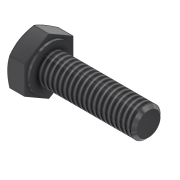
# Autodesk Inventor part: Sechskantschraube ISO 4017-M6x20-8.8
Saved by Autodesk Inventor 2015 (Build 190159000, 159)
## iProperties
Created: 2012-06-21
Part Number: Sechskantschraube ISO 4017-M6x20-8.8
Material: Steel
Document SubType Name: Modeling
Mass: 7.03009 g
Surface Area: 6.76348 cm^2
Volume: 0.895553 cm^3
Density: 7.85 g/cm^3
Appearance: Steel Galvanized 2
Autodesk Inventor part; units mm, degrees
ref_plane "YZ Plane" through (0, 0, 0) normal (1, 0, 0) x (0, 1, 0)
ref_plane "XZ Plane" through (0, 0, 0) normal (0, 1, 0) x (-1, 0, 0)
ref_plane "XY Plane" through (0, 0, 0) normal (0, 0, 1) x (1, 0, 0)
sketch "Sketch1" plane through (0, 0, 0) normal (0, 0, 1) x (1, 0, 0)
  line L0 (-8.8, 0) -> (24.8, 0) projected
  line L1 (20, 0) -> (20, 2.385)
  line L2 (20, 2.385) -> (19.385, 3)
  line L3 (19.385, 3) -> (0, 3)
  line L4 (0, 3) -> (0, 4.45)
  line L5 (0, 4.45) -> (-0.5, 4.45)
  line L6 (-0.5, 4.45) -> (-0.5, 5)
  line L7 (-0.5, 5) -> (-4, 5)
  line L8 (-4, 5) -> (-4, 0)
  point P0 (0, 0)
  dimension "d0" = 6
  dimension "d1" = 20
  dimension "d2" = 10
  dimension "d3" = 8.9
  dimension "d4" = 4
  dimension "d5" = 45
  dimension "d6" = 4.77
  dimension "d7" = 0.5
  constraints: 16 end point, 4 parallel, 3 perpendicular, 2 point on line, 1 vertical alignment
  measures "d0" diameter of L3 L0
  measures "d1" distance between parallel lines of L4 L1
  measures "d2" diameter of L7 L0
  measures "d3" diameter of L5 L0
  measures "d4" distance between parallel lines of L8 L4
  measures "d5" angle of L1 L2
  measures "d6" diameter of L1.end L0
  measures "d7" distance of L4.end L5.end
revolve "Revolution1" add sketch "Sketch1" angle 360 about axis through (-10, 0, 0) along (1, 0, 0)
sketch "Sketch2" plane through (-4, 0, 0) normal (-1, 0, 0) x (0, 0, 1)
  circle A0 centre (0, 0) radius 5 projected
  line L0 (2.8868, 5) -> (5.7735, 0)
  line L1 (5.7735, 0) -> (2.8868, -5)
  line L2 (2.8868, -5) -> (-2.8868, -5)
  line L3 (-2.8868, -5) -> (-5.7735, 0)
  line L4 (-5.7735, 0) -> (-2.8868, 5)
  line L5 (-2.8868, 5) -> (2.8868, 5)
  point P0 (0, 5)
  constraints: 12 end point, 2 vertical alignment, 1 coincident, 1 midpoint, 14 other
extrude "Extrusion1" add sketch "Sketch2" against normal up to surface (3.5 mm away)
sketch "Sketch3" plane through (0, 0, 0) normal (0, 0, 1) x (1, 0, 0)
  line L0 (-4, 5.55) -> (-0.5, 5.55)
  line L1 (-0.5, 5.55) -> (-0.5, 6.66)
  line L2 (-0.5, 6.66) -> (-4, 6.66)
  line L3 (-4, 6.66) -> (-4, 5.55)
  line L4 (-4.8, 0) -> (0.8, 0) projected
  line L5 (-4, 5) -> (-3.0416, 6.66)
  line L6 (-4, 5.55) -> (-4, 5)
  point P0 (0, 0)
  point P1 (-0.5, 5)
  dimension "d11" = 11.1
  dimension "d12" = 1.11
  dimension "d13" = 30
  constraints: 12 end point, 2 parallel, 2 perpendicular, 2 vertical alignment, 1 horizontal, 1 point on line
  measures "d11" diameter of L0 L4
  measures "d12" distance of L2.end L0.start
  measures "d13" angle of L6 L5
revolve "Revolution2" cut sketch "Sketch3" angle 360 about axis through (-10, 0, 0) along (1, 0, 0) contours L3 L2 L5 L0 | L0 L5 L6
thread "Thread1" size "M6x1" class "6g" standard "ISO Metric profile" full length
sketch "Sketch4" plane through (-4, 0, 0) normal (-1, 0, 0) x (0, 0, 1)
  circle A0 centre (0, 0) radius 3.75 construction
  spline S0 degree 2 poles (-2.4547, -1.0741) (-2.3544, -1.2038) (-2.112, -1.282) (-1.9755, -1.2387) knots 0 0 0 1 2 2 2
  spline S1 degree 2 poles (-1.9755, -1.2387) (-1.7677, -1.1728) (-1.5794, -0.7835) (-1.6577, -0.5365) knots 0 0 0 1 2 2 2
  spline S2 degree 2 poles (-1.6577, -0.5365) (-1.7371, -0.2866) (-2.1226, -0.0747) (-2.3304, -0.1406) knots 0 0 0 1 2 2 2
  spline S3 degree 2 poles (-2.3304, -0.1406) (-2.4626, -0.1826) (-2.6145, -0.3843) (-2.623, -0.5438) knots 0 0 0 1 2 2 2
  spline S4 degree 2 poles (-2.623, -0.5438) (-2.736, -0.3845) (-3.0498, -0.2826) (-3.227, -0.3389) knots 0 0 0 1 2 2 2
  spline S5 degree 2 poles (-3.227, -0.3389) (-3.4711, -0.4163) (-3.6941, -0.8677) (-3.6047, -1.1496) knots 0 0 0 1 2 2 2
  spline S6 degree 2 poles (-3.6047, -1.1496) (-3.5152, -1.4315) (-3.0713, -1.6712) (-2.8214, -1.5919) knots 0 0 0 1 2 2 2
  spline S7 degree 2 poles (-2.8214, -1.5919) (-2.6354, -1.5329) (-2.444, -1.2642) (-2.4547, -1.0741) knots 0 0 0 1 2 2 2
  spline S8 degree 2 poles (-2.8994, -1.3512) (-2.9996, -1.383) (-3.217, -1.348) (-3.3792, -1.1948) (-3.4133, -1.0873) knots 0 0 0 1 2 3 3 3
  spline S9 degree 2 poles (-3.4133, -1.0873) (-3.4668, -0.9187) (-3.319, -0.6335) (-3.1534, -0.581) knots 0 0 0 1 2 2 2
  spline S10 degree 2 poles (-3.1534, -0.581) (-2.9834, -0.527) (-2.6915, -0.6807) (-2.638, -0.8492) knots 0 0 0 1 2 2 2
  spline S11 degree 2 poles (-2.638, -0.8492) (-2.5855, -1.0149) (-2.7352, -1.2991) (-2.8994, -1.3512) knots 0 0 0 1 2 2 2
  spline S12 degree 2 poles (-2.0433, -0.9947) (-2.1784, -1.0376) (-2.4047, -0.9191) (-2.4486, -0.7811) knots 0 0 0 1 2 2 2
  spline S13 degree 2 poles (-2.4486, -0.7811) (-2.4914, -0.646) (-2.3759, -0.4206) (-2.2524, -0.3814) knots 0 0 0 1 2 2 2
  spline S14 degree 2 poles (-2.2524, -0.3814) (-2.1245, -0.3408) (-1.8929, -0.4608) (-1.8509, -0.593) knots 0 0 0 1 2 2 2
  spline S15 degree 2 poles (-1.8509, -0.593) (-1.808, -0.7282) (-1.9242, -0.9569) (-2.0433, -0.9947) knots 0 0 0 1 2 2 2
  line L0 (-3.75, -0.1349) -> (-3.471, -0.1349)
  line L1 (-3.471, -0.1349) -> (-3.471, 0.1441)
  line L2 (-3.471, 0.1441) -> (-3.75, 0.1441)
  line L3 (-3.75, 0.1441) -> (-3.75, -0.1349)
  spline S16 degree 2 poles (-2.6249, 0.538) (-2.6177, 0.3742) (-2.4648, 0.1705) (-2.3282, 0.1272) knots 0 0 0 1 2 2 2
  spline S17 degree 2 poles (-2.3282, 0.1272) (-2.1205, 0.0612) (-1.7421, 0.2706) (-1.6637, 0.5176) knots 0 0 0 1 2 2 2
  spline S18 degree 2 poles (-1.6637, 0.5176) (-1.5844, 0.7675) (-1.7772, 1.163) (-1.985, 1.2289) knots 0 0 0 1 2 2 2
  spline S19 degree 2 poles (-1.985, 1.2289) (-2.1172, 1.2709) (-2.3576, 1.1936) (-2.4566, 1.0683) knots 0 0 0 1 2 2 2
  spline S20 degree 2 poles (-2.4566, 1.0683) (-2.457, 1.2636) (-2.6546, 1.5278) (-2.8319, 1.5841) knots 0 0 0 1 2 2 2
  spline S21 degree 2 poles (-2.8319, 1.5841) (-3.076, 1.6615) (-3.5184, 1.4213) (-3.6079, 1.1394) knots 0 0 0 1 2 2 2
  spline S22 degree 2 poles (-3.6079, 1.1394) (-3.6973, 0.8576) (-3.4729, 0.4057) (-3.223, 0.3264) knots 0 0 0 1 2 2 2
  spline S23 degree 2 poles (-3.223, 0.3264) (-3.037, 0.2674) (-2.7257, 0.3765) (-2.6249, 0.538) knots 0 0 0 1 2 2 2
  spline S24 degree 2 poles (-3.1479, 0.568) (-3.2482, 0.5999) (-3.4056, 0.7538) (-3.4498, 0.9725) (-3.4156, 1.08) knots 0 0 0 1 2 3 3 3
  spline S25 degree 2 poles (-3.4156, 1.08) (-3.3621, 1.2486) (-3.0769, 1.3963) (-2.9113, 1.3438) knots 0 0 0 1 2 2 2
  spline S26 degree 2 poles (-2.9113, 1.3438) (-2.7413, 1.2898) (-2.5915, 0.996) (-2.645, 0.8274) knots 0 0 0 1 2 2 2
  spline S27 degree 2 poles (-2.645, 0.8274) (-2.6975, 0.6618) (-2.9837, 0.5159) (-3.1479, 0.568) knots 0 0 0 1 2 2 2
  spline S28 degree 2 poles (-2.243, 0.3656) (-2.3781, 0.4085) (-2.4947, 0.6358) (-2.4509, 0.7738) knots 0 0 0 1 2 2 2
  spline S29 degree 2 poles (-2.4509, 0.7738) (-2.408, 0.909) (-2.1836, 1.0265) (-2.0601, 0.9873) knots 0 0 0 1 2 2 2
  spline S30 degree 2 poles (-2.0601, 0.9873) (-1.9322, 0.9467) (-1.8122, 0.7151) (-1.8542, 0.5829) knots 0 0 0 1 2 2 2
  spline S31 degree 2 poles (-1.8542, 0.5829) (-1.897, 0.4477) (-2.1238, 0.3278) (-2.243, 0.3656) knots 0 0 0 1 2 2 2
  dimension "d17" = 7.5
  constraints: 1 centre point, 1 coincident, 1 other
  measures "d17" diameter of A0
extrude "Extrusion2" add sketch "Sketch4" along normal blind 0.1
equation "\"d7\" = 0.125 * d4"
equation "\"d12\" = 0.1 * d11"
body "Solid1"
